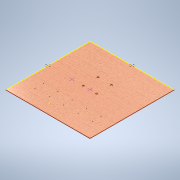
# Autodesk Inventor part: фанера
Saved by Autodesk Inventor 2020.1 (Build 241239000, 239)
## iProperties
Created: 2021-10-28
Part Number: фанера
Material: Древесина (дуб)
Document SubType Name: Modeling
Designer: Ni3na
Density: 0.76 g/cm^3
Appearance: Белый дуб — натуральный — с умеренным глянцем
Author: Ni3na
Autodesk Inventor part; units mm, degrees
ref_plane "YZ Plane" through (0, 0, 0) normal (1, 0, 0) x (0, 1, 0)
ref_plane "XZ Plane" through (0, 0, 0) normal (0, 1, 0) x (-1, 0, 0)
ref_plane "XY Plane" through (0, 0, 0) normal (0, 0, 1) x (1, 0, 0)
sketch "Эскиз1" plane through (0, 0, 0) normal (0, 1, 0) x (-1, 0, 0)
  line L0 (157.9407, 48.2001) -> (-242.0593, 48.2001)
  line L1 (-242.0593, 48.2001) -> (-242.0593, -351.7999)
  line L2 (-242.0593, -351.7999) -> (157.9407, -351.7999)
  line L3 (157.9407, -351.7999) -> (157.9407, 48.2001)
  point P0 (0, 0)
  dimension "d0" = 400
  dimension "d1" = 400
  constraints: 8 end point, 2 parallel, 1 horizontal, 1 perpendicular
  measures "d0" distance of L1.end L2.end
  measures "d1" distance of L0.end L1.end
extrude "Выдавливание1" add sketch "Эскиз1" along normal blind 2
sketch "Эскиз2" plane through (0, 2, 0) normal (0, 1, 0) x (1, 0, 0)
  line L0 (-157.9407, 351.7999) -> (-157.9407, -48.2001) projected
  line L1 (242.0593, 351.7999) -> (-157.9407, 351.7999) projected
  point P0 (0, 0)
  point P1 (-157.9407, 151.7999)
  point P2 (42.0593, 351.7999)
  point P3 (42.0593, 151.7999)
  point P4 (42.0593, 151.7999)
  point P5 (-44.4271, 151.7999)
  constraints: 2 midpoint, 1 coincident
sketch "Эскиз6" plane through (0, 0, 0) normal (0, -1, 0) x (1, 0, 0)
  line L0 (242.0593, -351.7999) -> (-157.9407, -351.7999) projected
  line L1 (-157.9407, -351.7999) -> (-157.9407, 48.2001) projected
  circle A0 centre (10.0593, -151.7939) radius 4
  circle A1 centre (42.0593, -186.9912) radius 47.5694
  circle A2 centre (74.0593, -151.7939) radius 4
  circle A3 centre (74.0593, -222.1885) radius 4
  circle A4 centre (10.0593, -222.1885) radius 4
  point P0 (0, 0)
  point P1 (42.0593, -351.7999)
  point P2 (-157.9407, -151.7999)
  point P3 (27.0149, -151.5386)
  dimension "d22" = 8
  dimension "d23" = 8
  dimension "d24" = 8
  dimension "d25" = 8
  dimension "d26" = 70.3946
  dimension "d27" = 64
  dimension "d28" = 70.3946
  dimension "d29" = 64
  constraints: 5 centre point, 4 point on circle, 2 coincident, 2 midpoint
  measures "d22" diameter of A0
  measures "d23" diameter of A2
  measures "d24" diameter of A3
  measures "d25" diameter of A4
  measures "d26" distance of A0.centre A4.centre
  measures "d27" distance of A0.centre A2.centre
  measures "d28" distance of A3.centre A2.centre
  measures "d29" distance of A4.centre A3.centre
extrude "Выдавливание3" cut sketch "Эскиз6" against normal blind 10 contours A0 A1 | A1 A0 | A2 A1 | A1 A2 | A4 A1 | A1 A4 | A3 A1 | A1 A3
sketch "Эскиз7" plane through (0, 0, 0) normal (0, -1, 0) x (1, 0, 0)
  circle A0 centre (178.7593, -26.7999) radius 1
  circle A1 centre (-94.4407, -26.7999) radius 1
  circle A2 centre (-26.1407, -26.7999) radius 1
  circle A3 centre (42.1593, -26.7999) radius 1
  circle A4 centre (110.4593, -26.7999) radius 1
  line L0 (242.0593, 48.2001) -> (242.0593, -351.7999) projected
  line L1 (-157.9407, 48.2001) -> (242.0593, 48.2001) projected
  circle A5 centre (178.7593, -66.7999) radius 1
  circle A6 centre (110.4593, -66.7999) radius 1
  circle A7 centre (42.0593, -66.7999) radius 1
  circle A8 centre (-26.1407, -66.7999) radius 1
  circle A9 centre (-94.4407, -66.7999) radius 1
  point P0 (0, 0)
  dimension "d33" = 2
  dimension "d34" = 2
  dimension "d35" = 2
  dimension "d36" = 2
  dimension "d37" = 2
  dimension "d38" = 63.3
  dimension "d39" = 75
  dimension "d40" = 68.3
  dimension "d41" = 68.3
  dimension "d42" = 68.3
  dimension "d43" = 68.3
  dimension "d44" = 2
  dimension "d45" = 2
  dimension "d46" = 2
  dimension "d47" = 2
  dimension "d48" = 40
  dimension "d49" = 40
  dimension "d50" = 40
  dimension "d51" = 40
  dimension "d52" = 40
  constraints: 10 centre point
  measures "d33" diameter of A0
  measures "d34" diameter of A1
  measures "d35" diameter of A2
  measures "d36" diameter of A3
  measures "d37" diameter of A4
  measures "d38" distance from line of A0.centre L0
  measures "d39" distance from line of L1 A0.centre
  measures "d40" distance of A4.centre A0.centre
  measures "d41" distance of A3.centre A4.centre
  measures "d42" distance of A2.centre A3.centre
  measures "d43" distance of A2.centre A1.centre
  measures "d44" diameter of A5
  measures "d45" diameter of A6
  measures "d46" diameter of A8
  measures "d47" diameter of A9
  measures "d48" distance of A0.centre A5.centre
  measures "d49" distance of A4.centre A6.centre
  measures "d50" vertical distance of A3.centre A7.centre
  measures "d51" distance of A2.centre A8.centre
  measures "d52" distance of A1.centre A9.centre
extrude "Выдавливание4" cut sketch "Эскиз7" against normal blind 10
